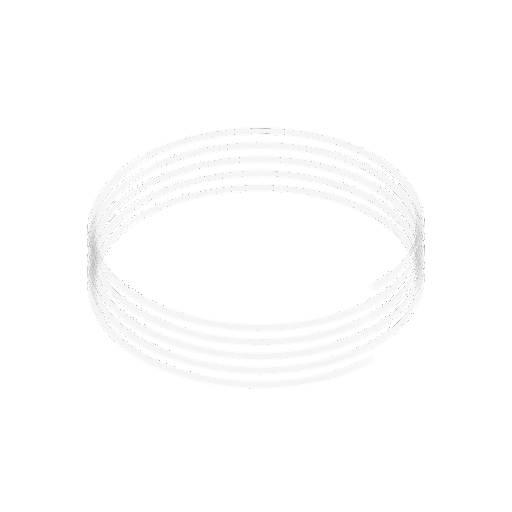
# Autodesk Inventor part: 00_Tube_Silicon_DI3mm_DO5mm
Saved by Autodesk Inventor 2024.1 (Build 281209000, 209)
## iProperties
Created: 2024-08-21
Part Number: 00_Tube_Silicon_DI3mm_DO5mm
Material: Generisch
Document SubType Name: Modeling
Designer: diederichbenedict
Density: 1 g/cm^3
Appearance: Polycarbonat - klar
Vendor: Amazon
Mass: 37.393 g
Surface Area: 748.164 cm^2
Volume: 37.393 cm^3
Author: diederichbenedict
Autodesk Inventor part; units mm, degrees
ref_plane "YZ Plane" through (0, 0, 0) normal (1, 0, 0) x (0, 1, 0)
ref_plane "XZ Plane" through (0, 0, 0) normal (0, 1, 0) x (-1, 0, 0)
ref_plane "XY Plane" through (0, 0, 0) normal (0, 0, 1) x (1, 0, 0)
sketch "Skizze1" plane through (0, 0, 0) normal (0, 1, 0) x (-1, 0, 0)
  circle A0 centre (0, 0) radius 1.5
  circle A1 centre (0, 0) radius 2.5
  line L0 (94.7175, 49.2125) -> (94.7175, -59.0026)
  dimension "d0" = 3
  dimension "d1" = 5
  constraints: 2 centre point, 2 coincident, 2 end point, 1 vertical
  measures "d0" diameter of A0
  measures "d1" diameter of A1
coil "Spirale1" sketch "Skizze1" operation add axis through (-94.7175, 0, 49.2125) along (0, 0, -1) pitch 10 turns 5 hand left
